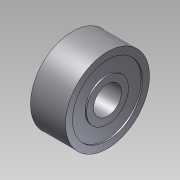
# Autodesk Inventor part: 2x6x2.5Bearing
Saved by Autodesk Inventor 2011 (Build 150239000, 239)
## iProperties
Created: 2011-02-22
Part Number: 2x6x2.5Bearing
Document SubType Name: Modeling
Designer: Casey
Density: 1 g/cm^3
Author: Casey
Autodesk Inventor part; units mm, degrees
ref_plane "YZ Plane" through (0, 0, 0) normal (1, 0, 0) x (0, 1, 0)
ref_plane "XZ Plane" through (0, 0, 0) normal (0, 1, 0) x (-1, 0, 0)
ref_plane "XY Plane" through (0, 0, 0) normal (0, 0, 1) x (1, 0, 0)
sketch "Sketch1" plane through (0, 0, 0) normal (0, 0, 1) x (1, 0, 0)
  line L0 (0.6114, 1) -> (1.25, 1)
  line L1 (1.25, 1) -> (1.25, 1.5)
  line L2 (1.25, 1.5) -> (1.15, 1.5)
  line L3 (1.15, 1.5) -> (1.15, 2.5)
  line L4 (1.15, 2.5) -> (1.25, 2.5)
  line L5 (1.25, 2.5) -> (1.25, 3)
  line L6 (1.25, 3) -> (-1.25, 3)
  line L7 (-1.25, 3) -> (-1.25, 2.5)
  line L8 (-1.25, 2.5) -> (-1.15, 2.5)
  line L9 (-1.15, 2.5) -> (-1.15, 1.5)
  line L10 (-1.15, 1.5) -> (-1.25, 1.5)
  line L11 (-1.25, 1.5) -> (-1.25, 1)
  line L12 (-1.25, 1) -> (0.6114, 1)
  line L13 (0, 0) -> (0, 3) construction
  line L14 (-1.75, 0) -> (1.75, 0) projected
  dimension "d0" = 0.1
  dimension "d1" = 1
  dimension "d2" = 0.5
  dimension "d3" = 2.5
  dimension "d4" = 3
  constraints: 28 end point, 9 parallel, 4 collinear, 4 equal length, 1 horizontal, 1 midpoint, 1 perpendicular, 1 vertical
  measures "d0" distance of L7.end L8.end
  measures "d1" vertical distance of L13.start L0.start
  measures "d2" distance of L10.end L11.end
  measures "d3" distance between parallel lines of L1 L11
  measures "d4" distance from line of L13.start L6
revolve "Revolution1" add sketch "Sketch1" angle 360 about axis through (-10, 0, 0) along (1, 0, 0)
body "Solid1"
